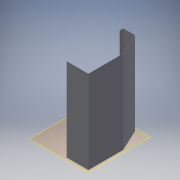
# Autodesk Inventor part: Back Cover
Saved by Autodesk Inventor 2018 (Build 220112000, 112)
## iProperties
Created: 2018-06-05
Part Number: Back Cover
Material: Generic
Document SubType Name: Modeling
Designer: P446509
Density: 1 g/cm^3
Appearance: Default
Author: P446509
Autodesk Inventor part; units mm, degrees
ref_plane "YZ Plane" through (0, 0, 0) normal (1, 0, 0) x (0, 1, 0)
ref_plane "XZ Plane" through (0, 0, 0) normal (0, 1, 0) x (-1, 0, 0)
ref_plane "XY Plane" through (0, 0, 0) normal (0, 0, 1) x (1, 0, 0)
ref_plane "Work Plane1" through (0, 0, 0) normal (0, 0, 1) x (1, 0, 0)
sketch "Sketch1" plane through (0, 0, 0) normal (0, 0, 1) x (1, 0, 0)
  line L0 (372.5286, -363.5164) -> (372.5286, 136.4836) projected
  line L1 (372.5286, 136.4836) -> (225.6417, 451.4836) projected
  line L2 (225.6417, 451.4836) -> (-104.3583, 451.4836) construction
  line L3 (-185.3519, -363.5164) -> (372.5286, -363.5164) construction
  line L4 (225.6417, 451.4836) -> (60.6417, 451.4836)
  line L5 (60.6417, 401.4836) -> (60.6417, 451.4836)
  line L6 (372.5286, -363.5164) -> (60.6417, -363.5164)
  line L7 (60.6417, 401.4836) -> (60.6417, -363.5164) construction
  line L8 (59.0417, 453.0836) -> (226.661, 453.0836)
  line L9 (226.661, 453.0836) -> (374.1286, 136.8383)
  line L10 (374.1286, 136.8383) -> (374.1286, -365.1164)
  line L11 (374.1286, -365.1164) -> (60.6417, -365.1164)
  line L12 (60.6417, -363.5164) -> (60.6417, -365.1164)
  line L13 (60.6417, 401.4836) -> (59.0417, 401.4836)
  line L14 (59.0417, 401.4836) -> (59.0417, 453.0836)
  point P0 (0, 0)
  dimension "d0" = 50
  dimension "d1" = 1.6
  dimension "d2" = 1.6
  dimension "d3" = 816.6
  dimension "d4" = 816.6
  constraints: 22 end point, 4 perpendicular, 2 parallel, 1 horizontal, 1 midpoint, 1 point on line, 1 other
  measures "d0" distance of L5.start L4.end
  measures "d1" distance between parallel lines of L0 L10
  measures "d2" distance of L5.start L13.end
  measures "d3" distance between parallel lines of L3 L8
  measures "d4" distance between parallel lines of L11 L2
extrude "Extrusion1" add sketch "Sketch1" along normal blind 1198.4 and the other way blind 1.6
sketch "Sketch2" plane through (59.0417, 401.4836, -1.6) normal (-1, 0, 0) x (0, 0, 1)
  line L0 (0, 0) -> (0, 51.6) projected
  line L1 (1200, 0) -> (0, 0) projected
  line L2 (0, 50) -> (0, 0)
  line L3 (0, 0) -> (1.6, 0)
  line L4 (1.6, 0) -> (1.6, 50)
  line L5 (0, 50) -> (1.6, 50) projected
  point P0 (1.6, -401.4836)
  point P1 (0, 50)
  dimension "d14" = 1.6
  constraints: 4 end point, 3 point on line, 2 parallel, 1 vertical, 3 other
  measures "d14" distance between parallel lines of L0 L4
extrude "Extrusion2" cut sketch "Sketch2" against normal blind 1.6
ref_plane "Work Plane2" through (0, 0, 598.4) normal (0, 0, 1) x (1, 0, 0)
mirror "Mirror1" about plane through (0, 0, 598.4) normal (0, 0, 1) of "Extrusion2"
body "Solid1"
